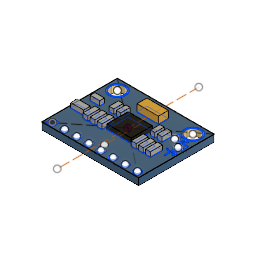
MPU_6050 (Autodesk Fusion 360 design; units mm, degrees)
Autodesk Fusion 360 part; units mm, degrees
note: some values were not read from the file. Set by a fixed rule: which sketch regions a step uses.
sketch "Sketch1" plane through (0, 0, 0) normal (0, 0, 1) x (1, 0, 0) in component "pcb"
  line L0 (10.25, -8) -> (-10.25, -8)
  line L1 (-10.25, -8) -> (-10.25, 8)
  line L2 (-10.25, 8) -> (10.25, 8)
  line L3 (10.25, 8) -> (10.25, -8)
  line L4 (10.25, -8) -> (-10.25, 8) construction
  line L5 (-10.25, -8) -> (10.25, 8) construction
  line L6 (0, 15) -> (0, -15) construction
  circle A0 centre (-8, 5.75) radius 1.5
  circle A1 centre (8, 5.75) radius 1.5
  circle A2 centre (-9, -7) radius 0.5
  circle A3 centre (-6.4286, -7) radius 0.5
  circle A4 centre (-3.8571, -7) radius 0.5
  circle A5 centre (-1.2857, -7) radius 0.5
  circle A6 centre (1.2857, -7) radius 0.5
  circle A7 centre (3.8571, -7) radius 0.5
  circle A8 centre (6.4286, -7) radius 0.5
  circle A9 centre (9, -7) radius 0.5
  line L7 (-2, 2) -> (3.2, 2)
  line L8 (3.2, 2) -> (3.2, -2.4975)
  line L9 (3.2, -2.4975) -> (-2, -2.4975)
  line L10 (-2, -2.4975) -> (-2, 2)
  line L11 (-2, 6) -> (2.5423, 6)
  line L12 (2.5423, 6) -> (2.5423, 3.8983)
  line L13 (2.5423, 3.8983) -> (-2, 3.8983)
  line L14 (-2, 3.8983) -> (-2, 6)
  circle A10 centre (-6.4286, -7) radius 0.75
  circle A11 centre (-3.8571, -7) radius 0.75
  circle A12 centre (-1.2857, -7) radius 0.75
  circle A13 centre (1.2857, -7) radius 0.75
  circle A14 centre (3.8571, -7) radius 0.75
  circle A15 centre (6.4286, -7) radius 0.75
  circle A16 centre (9, -7) radius 0.75
  circle A17 centre (-8, 5.75) radius 1.75
  circle A18 centre (8, 5.75) radius 1.75
  line L15 (-9.7685, -2.4026) -> (-7, -2.4026)
  line L16 (-7, -2.4026) -> (-7, -1)
  line L17 (-7, -1) -> (-9.7685, -1)
  line L18 (-9.7685, -1) -> (-9.7685, -2.4026)
  line L19 (-9, 2) -> (-7, 2)
  line L20 (-7, 2) -> (-7, 1)
  line L21 (-7, 1) -> (-9, 1)
  line L22 (-9, 1) -> (-9, 2)
  line L23 (-5, 3) -> (-4, 3)
  line L24 (-4, 3) -> (-4, 1)
  line L25 (-4, 1) -> (-5, 1)
  line L26 (-5, 1) -> (-5, 3)
  line L27 (-2.5468, 3) -> (-3.4677, 3)
  line L28 (-3.4677, 3) -> (-3.4677, 1)
  line L29 (-3.4677, 1) -> (-2.5468, 1)
  line L30 (-2.5468, 1) -> (-2.5468, 3)
  line L31 (-6.5365, -0.4638) -> (-5.5, -0.4638)
  line L32 (-5.5, -0.4638) -> (-5.5, -3)
  line L33 (-5.5, -3) -> (-6.5365, -3)
  line L34 (-6.5365, -3) -> (-6.5365, -0.4638)
  line L35 (-5.0365, -3) -> (-5.0365, -0.4638)
  line L36 (-5.0365, -0.4638) -> (-4, -0.4638)
  line L37 (-4, -3) -> (-5.0365, -3)
  line L38 (-4, -0.4638) -> (-4, -3)
  line L39 (-3.5365, -3) -> (-3.5365, -0.4638)
  line L40 (-3.5365, -0.4638) -> (-2.5, -0.4638)
  line L41 (-2.5, -3) -> (-3.5365, -3)
  line L42 (-2.5, -0.4638) -> (-2.5, -3)
  line L43 (0.6, 2) -> (0.6, -5.5829) construction
  line L44 (4.6676, 1) -> (3.7468, 1)
  line L45 (3.7468, 1) -> (3.7468, 3)
  line L46 (4.6676, 3) -> (4.6676, 1)
  line L47 (3.7468, 3) -> (4.6676, 3)
  line L48 (5.2, 1) -> (6.2, 1)
  line L49 (6.2, 1) -> (6.2, 3)
  line L50 (5.2, 3) -> (5.2, 1)
  line L51 (6.2, 3) -> (5.2, 3)
  line L52 (5.2, -3) -> (6.2364, -3)
  line L53 (6.2364, -3) -> (6.2364, -0.4638)
  line L54 (5.2, -0.4638) -> (5.2, -3)
  line L55 (6.2364, -0.4638) -> (5.2, -0.4638)
  line L56 (6.7, -3) -> (7.7364, -3)
  line L57 (7.7364, -3) -> (7.7364, -0.4638)
  line L58 (6.7, -0.4638) -> (6.7, -3)
  line L59 (7.7364, -0.4638) -> (6.7, -0.4638)
  line L60 (3.7, -3) -> (4.7364, -3)
  line L61 (4.7364, -3) -> (4.7364, -0.4638)
  line L62 (3.7, -0.4638) -> (3.7, -3)
  line L63 (4.7364, -0.4638) -> (3.7, -0.4638)
  line L64 (-8.25, -6.25) -> (-9.75, -6.25)
  line L65 (-9.75, -6.25) -> (-9.75, -7.75)
  line L66 (-9.75, -7.75) -> (-8.25, -7.75)
  line L67 (-8.25, -7.75) -> (-8.25, -6.25)
  line L68 (-8.25, -6.25) -> (-9.75, -7.75) construction
  line L69 (-9.75, -6.25) -> (-8.25, -7.75) construction
  arc A19 (-9.5792, -7.4765) -> (-9.5303, -7.5303) centre (-9, -7) ccw
  line L70 (9.8, 2.8) -> (9.8, 3)
  line L71 (7, 2.9988) -> (7, 2.8021)
  line L72 (7, 2.8021) -> (7.4945, 2.3076)
  line L73 (7.4945, 2.3076) -> (7.6359, 2.4491)
  line L74 (7.284, 3) -> (7.6366, 3.3525)
  line L75 (7.6366, 3.3525) -> (7.4951, 3.494)
  line L76 (7.4951, 3.494) -> (7.0002, 2.999)
  line L77 (7.6359, 2.4491) -> (7.285, 2.8)
  line L78 (7.0002, 2.999) -> (7, 2.9988)
  line L79 (9.0312, 3.7918) -> (8.3787, 3.9666)
  line L80 (8.5401, 3.7163) -> (8.9795, 3.5986)
  line L81 (8.9795, 3.5986) -> (9.0312, 3.7918)
  line L82 (8.2028, 3.8607) -> (8.0939, 3.2434)
  line L83 (8.0939, 3.2434) -> (8.2909, 3.2087)
  line L84 (8.3787, 3.9666) -> (8.2028, 3.8607)
  line L85 (8.2909, 3.2087) -> (8.3637, 3.6214)
  line L86 (8.2266, 1.9652) -> (8.3859, 1.8438)
  line L87 (7.285, 2.8) -> (8.5392, 2.8)
  line L88 (8.7399, 2.8) -> (9.8, 2.8)
  arc A20 (8.2266, 1.9652) -> (8.5392, 2.8) centre (7, 2.9005) ccw
  arc A21 (8.5393, 3) -> (8.3637, 3.6214) centre (7, 2.9005) ccw
  line L89 (9.8, 3) -> (8.74, 3)
  line L90 (8.5393, 3) -> (7.284, 3)
  arc A22 (8.3859, 1.8438) -> (8.7399, 2.8) centre (7, 2.9005) ccw
  arc A23 (8.74, 3) -> (8.5401, 3.7163) centre (7, 2.9005) ccw
  line L91 (8.7766, 1.4388) -> (8.7766, 0.1845)
  line L92 (8.4257, 1.0878) -> (8.7766, 1.4388)
  line L93 (8.2843, 1.2292) -> (8.4257, 1.0878)
  line L94 (8.7788, 1.7237) -> (8.2843, 1.2292)
  line L95 (8.9755, 1.7237) -> (8.7788, 1.7237)
  line L96 (8.9756, 1.7236) -> (8.9755, 1.7237)
  line L97 (9.4706, 1.2286) -> (8.9756, 1.7236)
  line L98 (9.3292, 1.0872) -> (9.4706, 1.2286)
  line L99 (8.9766, 1.4397) -> (9.3292, 1.0872)
  line L100 (8.9766, 0.1844) -> (8.9766, 1.4397)
  arc A24 (8.9766, 0.1844) -> (9.598, 0.3601) centre (8.8771, 1.7237) ccw
  line L101 (9.1853, 0.4329) -> (9.598, 0.3601)
  line L102 (9.22, 0.6298) -> (9.1853, 0.4329)
  line L103 (9.8373, 0.521) -> (9.22, 0.6298)
  line L104 (9.9432, 0.3451) -> (9.8373, 0.521)
  line L105 (9.7684, -0.3075) -> (9.9432, 0.3451)
  line L106 (9.5752, -0.2557) -> (9.7684, -0.3075)
  line L107 (9.6929, 0.1837) -> (9.5752, -0.2557)
  arc A25 (8.9766, -0.0162) -> (9.6929, 0.1837) centre (8.8771, 1.7237) ccw
  line L108 (8.9766, -1.0763) -> (8.9766, -0.0162)
  line L109 (8.7766, -1.0763) -> (8.9766, -1.0763)
  line L110 (8.7766, -0.0162) -> (8.7766, -1.0763)
  arc A26 (7.8204, 0.3378) -> (8.7766, -0.0162) centre (8.8771, 1.7237) ccw
  line L111 (7.9419, 0.4971) -> (7.8204, 0.3378)
  arc A27 (7.9419, 0.4971) -> (8.7766, 0.1845) centre (8.8771, 1.7237) ccw
  line L112 (6.5, 3.5) -> (6.8, 3.8)
  line L113 (6.8, 3.8) -> (6.5, 4.1)
  line L114 (6.5, 4.1) -> (6.65, 4.25)
  line L115 (6.65, 4.25) -> (7, 3.9)
  line L116 (7, 3.7) -> (6.65, 3.35)
  line L117 (6.5, 3.5) -> (6.65, 3.35)
  line L118 (7, 3.7) -> (7.4, 3.7)
  line L119 (7.4, 3.7) -> (7.4, 3.9)
  line L120 (7.4, 3.9) -> (7, 3.9)
  line L121 (6.5, 4.1) -> (6.65, 4.25)
  line L122 (6.65, 4.25) -> (7, 3.9)
  line L123 (7.4, 3.9) -> (7, 3.9)
  line L124 (7.4, 3.7) -> (7.4, 3.9)
  line L125 (7, 3.7) -> (7.4, 3.7)
  line L126 (7, 3.7) -> (6.65, 3.35)
  line L127 (6.5, 3.5) -> (6.65, 3.35)
  line L128 (6.5, 3.5) -> (6.8, 3.8)
  line L129 (6.8, 3.8) -> (6.5, 4.1)
  line L130 (9.22, 2.1903) -> (9.37, 2.3403)
  line L131 (9.37, 2.3403) -> (9.67, 2.0403)
  line L132 (9.67, 1.7403) -> (9.37, 1.4403)
  line L133 (9.22, 1.5903) -> (9.37, 1.4403)
  line L134 (9.22, 1.5903) -> (9.52, 1.8903)
  line L135 (9.52, 1.8903) -> (9.22, 2.1903)
  line L136 (9.67, 2.0403) -> (9.97, 2.3403)
  line L137 (10.12, 2.1903) -> (9.97, 2.3403)
  line L138 (10.12, 2.1903) -> (9.82, 1.8903)
  line L139 (9.82, 1.8903) -> (10.12, 1.5903)
  line L140 (10.12, 1.5903) -> (9.97, 1.4403)
  line L141 (9.97, 1.4403) -> (9.67, 1.7403)
  point P0 (-9, -7)
  dimension "d1" = 20.5
  dimension "d2" = 16
  dimension "d3" = 3
  dimension "d4" = 8
  dimension "d6" = 2.25
  dimension "d7" = 1
  dimension "d10" = 18
  dimension "d11" = 0
  dimension "d12" = 1.5
  dimension "d17" = 3.5
  dimension "d18" = 3.5
  dimension "d21" = 3
  dimension "d22" = 0
  dimension "d33" = 1.5
  dimension "d34" = 1.5
  constraint perpendicular L0 L1
  constraint parallel L0 L2
  constraint parallel L1 L3
  constraint horizontal L0
  constraint coincident L4 origin
  constraint coincident L5 origin
  constraint perpendicular L0 L6
  constraint symmetric L6 A0 A1
  constraint horizontal L7
  constraint vertical L8
  constraint horizontal L9
  constraint vertical L10
  constraint coincident L4 L8.end
  constraint horizontal L11
  constraint vertical L12
  constraint horizontal L13
  constraint vertical L14
  constraint concentric A2 A19
  constraint concentric A0 A17
  constraint concentric A1 A18
  constraint horizontal L15
  constraint vertical L16
  constraint horizontal L17
  constraint vertical L18
  constraint horizontal L19
  constraint vertical L20
  constraint horizontal L21
  constraint vertical L22
  constraint horizontal L23
  constraint vertical L24
  constraint horizontal L25
  constraint vertical L26
  constraint horizontal L27
  constraint vertical L28
  constraint horizontal L29
  constraint vertical L30
  constraint horizontal L31
  constraint vertical L32
  constraint horizontal L33
  constraint vertical L34
  constraint midpoint L7 L43.start
  constraint perpendicular L7 L43
  constraint symmetric L23.start L43 L49.end
  constraint symmetric L23.end L43 L50.start
  constraint symmetric L24.end L43 L48.start
  constraint symmetric L25.end L43 L48.end
  constraint symmetric L27.start L43 L45.end
  constraint symmetric L27.end L43 L46.start
  constraint symmetric L28.end L43 L44.start
  constraint symmetric L29.end L43 L44.end
  constraint symmetric L31.start L43 L57.end
  constraint symmetric L31.end L43 L58.start
  constraint symmetric L32.end L43 L56.start
  constraint symmetric L33.end L43 L56.end
  constraint symmetric L35.start L43 L52.end
  constraint symmetric L35.end L43 L53.end
  constraint symmetric L36.end L43 L54.start
  constraint symmetric L37.start L43 L52.start
  constraint symmetric L39.start L43 L60.end
  constraint symmetric L39.end L43 L61.end
  constraint symmetric L40.end L43 L62.start
  constraint symmetric L41.start L43 L60.start
  constraint perpendicular L64 L65
  constraint parallel L64 L66
  constraint parallel L65 L67
  constraint horizontal L64
  constraint coincident L68 P0
  constraint coincident L69 P0
  constraint coincident P0 A2.centre
  constraint coincident L5 A19.start
  constraint coincident L68 A19.end
  constraint vertical L70
  constraint horizontal L89
  constraint vertical L71
  constraint parallel L76 L78
  constraint collinear L87 L88
  constraint coincident A21.start L89
  constraint concentric A20 A21
  constraint coincident L89.end A22
  constraint collinear L89 L90
  constraint concentric A22 A23
  constraint parallel L96 L97
  constraint collinear L91 L110
  constraint coincident L100.start L108
  constraint concentric A24 A27
  constraint coincident A25.start A26
  constraint collinear L100 L108
  constraint concentric A25 A26
  constraint perpendicular L112 L113
  constraint perpendicular L113 L114
  constraint perpendicular L114 L115
  constraint perpendicular L115 L116
  constraint perpendicular L116 L117
  constraint horizontal L118
  constraint perpendicular L118 L119
  constraint perpendicular L119 L120
  constraint perpendicular L128 L129
  constraint perpendicular L121 L129
  constraint perpendicular L121 L122
  constraint perpendicular L122 L126
  constraint perpendicular L126 L127
  constraint horizontal L125
  constraint perpendicular L124 L125
  constraint perpendicular L123 L124
  constraint perpendicular L134 L135
  constraint perpendicular L130 L135
  constraint perpendicular L130 L131
  constraint perpendicular L131 L132
  constraint perpendicular L132 L133
  constraint perpendicular L138 L139
  constraint perpendicular L139 L140
  constraint perpendicular L140 L141
  constraint perpendicular L136 L141
  constraint perpendicular L136 L137
  measures "d1" distance of L1.end L2.end
  measures "d2" distance of L0.end L1.end
  measures "d3" diameter of A0
  measures "d4" distance of L6 A0.centre
  measures "d6" distance of L2 A0.centre
  measures "d7" diameter of A2
  measures "d12" diameter of A19
  measures "d17" diameter of A17
  measures "d18" diameter of A18
  measures "d33" distance of L64.end L65.end
  measures "d34" distance of L65.end L66.end
extrude "Extrude1" add sketch "Sketch1" against normal blind 1.5 contours L0 L1 L2 L3 | A0 | A1 | A2 | A3 | A4 | A5 | A6 | A7 | A8 | A9 | L7 L8 L9 L10 | L11 L12 L13 L14 | A10 | A11 | A12 | A13 | A14 | A15 | A16 | A17 | A18 | L15 L16 L17 L18 | L19 L20 L21 L22 | L23 L24 L25 L26 | L27 L28 L29 L30 | L31 L32 L33 L34 | L35 L36 L37 L38 | L39 L40 L41 L42 | L44 L45 L46 L47 | L48 L49 L50 L51 | L52 L53 L54 L55 | L56 L57 L58 L59 | L60 L61 L62 L63 | L64 L65 L66 L67 | L70 L71 L72 L73 L74 L75 L76 L77 L79 L80 L81 L82 L83 L84 L85 L86 L87 L88 A20 A21 L89 L90 A22 A23 | L91 L92 L93 L94 L95 L97 L98 L99 L100 A24 L101 L102 L103 L104 L105 L106 L107 A25 L108 L109 L110 A26 L111 A27 | L112 L113 L114 L115 L116 L117 L118 L119 L120 L121 L122 L123 L124 L125 L126 L127 L128 L129 | L130 L131 L132 L133 L134 L135 L136 L137 L138 L139 L140 L141 makes body 1 in component "pcb"
extrude "Extrude2" cut sketch "Sketch1" against normal blind 2 contours A0 | A1 | A2 | A3 | A4 | A5 | A6 | A7 | A8 | A9 bodies 1 in component "pcb"
extrude "Extrude3" add sketch "Sketch1" along normal blind 1 separate body contours L7 L8 L9 L10 makes body 2 in component "pcb"
extrude "Extrude4" add sketch "Sketch1" along normal blind 1.5 separate body contours L11 L12 L13 L14 makes body 3 in component "pcb"
extrude "Extrude5" add sketch "Sketch1" along normal blind 1 separate body contours L15 L16 L17 L18 | L19 L20 L21 L22 | L23 L24 L25 L26 | L27 L28 L29 L30 | L31 L32 L33 L34 | L35 L36 L37 L38 | L39 L40 L41 L42 | L44 L45 L46 L47 | L48 L49 L50 L51 | L52 L53 L54 L55 | L56 L57 L58 L59 | L60 L61 L62 L63 makes body 4 at (-6.191, -1.3092, 0) makes body 5 at (-2.5468, 1.6667, 0.3333) makes body 6 at (5.5333, 2.3333, 0) makes body 7 at (5.8909, -2.1546, 0) makes body 8 at (-4.6667, 2.3333, 0) makes body 9 at (-8.3333, 1.6667, 0) makes body 10 at (-3.191, -1.3092, 0) makes body 11 at (7.0454, -1.3092, 0) makes body 12 at (3.7468, 1.6667, 0.3333) makes body 13 at (4.0454, -1.3092, 0) makes body 14 at (-4.691, -1.3092, 0) makes body 15 at (-7.9228, -1.935, 0) in component "pcb"
extrude "Extrude6" cut sketch "Sketch1" against normal blind 3 contours A10 | A11 | A12 | A13 | A14 | A15 | A16 | A17 | A18 | L64 L65 L66 L67 bodies 1 in component "pcb"
extrude "Extrude7" add sketch "Sketch1" against normal up to surface (1.5 mm away) separate body contours A10 | A11 | A12 | A13 | A14 | A15 | A16 | A17 | A18 | L64 L65 L66 L67 makes body 16 at (9.7491, -7.0374, -1) makes body 17 at (-0.5366, -7.0374, -1) makes body 18 at (-8.5006, -7.0249, -1) makes body 19 at (2.0348, -7.0374, -1) makes body 20 at (-6.2522, 5.6628, -1) makes body 21 at (7.1776, -7.0374, -1) makes body 22 at (-3.1081, -7.0374, -1) makes body 23 at (-5.6795, -7.0374, -1) makes body 24 at (4.6062, -7.0374, -1) makes body 25 at (9.7478, 5.6628, -1) in component "pcb"
extrude "Extrude8" cut sketch "Sketch1" against normal blind 0.5 contours L70 L71 L72 L73 L74 L75 L76 L77 L79 L80 L81 L82 L83 L84 L85 L86 L87 L88 A20 A21 L89 L90 A22 A23 | L91 L92 L93 L94 L95 L97 L98 L99 L100 A24 L101 L102 L103 L104 L105 L106 L107 A25 L108 L109 L110 A26 L111 A27 | L112 L113 L114 L115 L116 L117 L118 L119 L120 L121 L122 L123 L124 L125 L126 L127 L128 L129 | L130 L131 L132 L133 L134 L135 L136 L137 L138 L139 L140 L141 bodies 1 in component "pcb"
extrude "Extrude9" add sketch "Sketch1" against normal blind 0.5 separate body contours L70 L71 L72 L73 L74 L75 L76 L77 L79 L80 L81 L82 L83 L84 L85 L86 L87 L88 A20 A21 L89 L90 A22 A23 | L91 L92 L93 L94 L95 L97 L98 L99 L100 A24 L101 L102 L103 L104 L105 L106 L107 A25 L108 L109 L110 A26 L111 A27 | L112 L113 L114 L115 L116 L117 L118 L119 L120 L121 L122 L123 L124 L125 L126 L127 L128 L129 | L130 L131 L132 L133 L134 L135 L136 L137 L138 L139 L140 L141 makes body 26 at (9.52, 1.6903, 0) makes body 27 at (7.7028, 2.9333, 0) makes body 28 at (8.91, 0.6029, 0) makes body 29 at (6.8167, 3.6167, 0) in component "pcb"
component "pcb" placed x (1, 0, 0) y (0, 1, 0) z (0, 0, 1) at (0, 0, 0)
